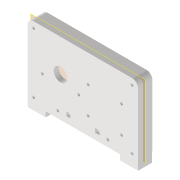
# Autodesk Inventor part: 10_Cassette_microscopy_deck
Saved by Autodesk Inventor 2022 (Build 260153000, 153)
## iProperties
Created: 2023-02-06
Part Number: 10_Cassette_microscopy_deck
Material: Generisch
Document SubType Name: Modeling
Designer: diederichbenedict
Density: 1 g/cm^3
Appearance: Vorgabe
Author: diederichbenedict
Autodesk Inventor part; units mm, degrees
ref_plane "YZ Plane" through (0, 0, 0) normal (1, 0, 0) x (0, 1, 0)
ref_plane "Arbeitsebene1" through (0, 0, 0) normal (0, 0, 1) x (1, 0, 0)
sketch "Skizze1" plane through (0, 0, 0) normal (0, 0, 1) x (1, 0, 0)
  line L0 (79.0515, 12.2449) -> (82.2341, -2.728) projected
  arc A0 (82.2417, -2.8) -> (82.2341, -2.728) centre (81.8953, -2.8001) ccw projected
  line L1 (82.2417, -2.8) -> (94.4, -2.8) projected
  arc A1 (94.4, -2.8) -> (97.2, 0) centre (94.4, 0) ccw projected
  line L2 (97.2, 0) -> (97.2, 57.5) projected
  arc A2 (97.2, 57.5) -> (94.4, 60.3) centre (94.4, 57.5) ccw projected
  line L3 (94.4, 60.3) -> (0, 60.3) projected
  arc A3 (0, 60.3) -> (-2.8, 57.5) centre (0, 57.5) ccw projected
  line L4 (-2.8, 57.5) -> (-2.8, 0) projected
  arc A4 (-2.8, 0) -> (0, -2.8) centre (0, 0) ccw projected
  line L5 (0, -2.8) -> (12.1583, -2.8) projected
  arc A5 (12.1659, -2.728) -> (12.1583, -2.8) centre (12.5047, -2.8001) ccw projected
  line L6 (12.1659, -2.728) -> (15.3485, 12.2449) projected
  spline S0 degree 3 poles (15.3485, 12.2449) (15.4002, 12.4886) (15.5255, 12.6991) (15.7047, 12.8442) (15.8839, 12.9893) (16.1159, 13.0681) (16.365, 13.0681) knots 2.565195 2.565195 2.565195 2.565195 3.141593 3.141593 3.141593 3.717991 3.717991 3.717991 3.717991 projected
  line L7 (16.365, 13.0681) -> (78.035, 13.0681) projected
  spline S1 degree 3 poles (78.035, 13.0681) (78.2841, 13.0681) (78.5161, 12.9893) (78.6953, 12.8442) (78.8745, 12.6991) (78.9998, 12.4886) (79.0515, 12.2449) knots 2.565195 2.565195 2.565195 2.565195 3.141593 3.141593 3.141593 3.717991 3.717991 3.717991 3.717991 projected
  circle A6 centre (47.2, 46) radius 2.3 projected
  line L8 (45.2128, 29.3892) -> (45.2128, 34.3892) projected
  line L9 (45.2128, 34.3892) -> (47.227, 34.3892) projected
  spline S2 degree 3 poles (47.227, 34.3892) (47.2755, 34.3889) (47.3689, 34.3884) (47.5045, 34.3868) (47.6304, 34.3823) (47.7467, 34.3783) (47.8531, 34.3692) (47.9503, 34.362) (48.0382, 34.3521) (48.1418, 34.3361) (48.2622, 34.3113) (48.3982, 34.2653) (48.5271, 34.2078) (48.647, 34.1347) (48.7582, 34.0492) (48.8617, 33.9521) (48.9526, 33.8392) (49.0345, 33.7161) (49.1036, 33.5825) (49.1512, 33.4389) (49.1816, 33.2877) (49.1853, 33.1841) (49.1872, 33.1312) knots 0 0 0 0 0.054831 0.105884 0.153553 0.197457 0.237653 0.274456 0.307946 0.337788 0.393117 0.446926 0.500064 0.552657 0.605522 0.658748 0.713023 0.769236 0.826057 0.882736 0.940135 1 1 1 1 projected
  spline S3 degree 3 poles (49.1872, 33.1312) (49.1852, 33.0736) (49.1814, 32.96) (49.1456, 32.7934) (49.0886, 32.6341) (49.0082, 32.4845) (48.9096, 32.3472) (48.7931, 32.2267) (48.6602, 32.1236) (48.5604, 32.0723) (48.5101, 32.0465) knots 0 0 0 0 0.127883 0.252157 0.376787 0.502926 0.628342 0.751132 0.874457 1 1 1 1 projected
  spline S4 degree 3 poles (48.5101, 32.0465) (48.544, 32.0349) (48.611, 32.0121) (48.7069, 31.9702) (48.7968, 31.9215) (48.8806, 31.8678) (48.959, 31.8084) (49.0295, 31.7416) (49.0964, 31.671) (49.1552, 31.5932) (49.2083, 31.5118) (49.2534, 31.4256) (49.2925, 31.3367) (49.3252, 31.2441) (49.3485, 31.1473) (49.3671, 31.0475) (49.3767, 30.9439) (49.3785, 30.8739) (49.3795, 30.8385) knots 0 0 0 0 0.067041 0.132557 0.19578 0.258217 0.318868 0.379478 0.440087 0.500739 0.561785 0.621919 0.682673 0.743576 0.805446 0.868975 0.933677 1 1 1 1 projected
  spline S5 degree 3 poles (49.3795, 30.8385) (49.3775, 30.782) (49.3735, 30.6692) (49.3435, 30.5009) (49.2928, 30.3355) (49.2242, 30.1742) (49.139, 30.0221) (49.0388, 29.8833) (48.9219, 29.7624) (48.7924, 29.656) (48.6465, 29.5678) (48.4843, 29.5001) (48.3069, 29.449) (48.1819, 29.432) (48.1175, 29.4233) knots 0 0 0 0 0.081255 0.162135 0.244884 0.329397 0.413636 0.495044 0.574817 0.654649 0.735398 0.818839 0.906654 1 1 1 1 projected
  spline S6 degree 3 poles (48.1175, 29.4233) (48.0928, 29.4212) (48.0361, 29.4164) (47.9399, 29.4104) (47.8217, 29.4059) (47.6815, 29.4006) (47.5189, 29.3968) (47.3342, 29.3942) (47.1272, 29.3908) (46.982, 29.3897) (46.9055, 29.3892) knots 0 0 0 0 0.061321 0.140766 0.238316 0.354022 0.487867 0.640687 0.810851 1 1 1 1 projected
  line L10 (46.9055, 29.3892) -> (45.2128, 29.3892) projected
  circle A7 centre (68.575, 31.8892) radius 6.4815 projected
  circle A8 centre (25.825, 31.8892) radius 6.4815 projected
  line L11 (44.025, 27.3892) -> (44.025, 15.8892) projected
  arc A9 (41.825, 13.6892) -> (44.025, 15.8892) centre (41.825, 15.8892) ccw projected
  line L12 (41.825, 13.6892) -> (9.825, 13.6892) projected
  arc A10 (7.625, 15.8892) -> (9.825, 13.6892) centre (9.825, 15.8892) ccw projected
  line L13 (7.625, 15.8892) -> (7.625, 47.8892) projected
  arc A11 (9.825, 50.0892) -> (7.625, 47.8892) centre (9.825, 47.8892) ccw projected
  line L14 (9.825, 50.0892) -> (41.825, 50.0892) projected
  arc A12 (44.025, 47.8892) -> (41.825, 50.0892) centre (41.825, 47.8892) ccw projected
  line L15 (44.025, 47.8892) -> (44.025, 36.3892) projected
  arc A13 (41.825, 34.1892) -> (44.025, 36.3892) centre (41.825, 36.3892) ccw projected
  line L16 (41.825, 34.1892) -> (33.4237, 34.1892) projected
  arc A14 (32.3338, 34.8872) -> (33.4237, 34.1892) centre (33.4237, 35.3892) ccw projected
  arc A15 (32.3338, 34.8872) -> (19.2006, 34.6222) centre (25.825, 31.8892) ccw projected
  arc A16 (18.5535, 34.1892) -> (19.2006, 34.6222) centre (18.5535, 34.8892) ccw projected
  line L17 (18.5535, 34.1892) -> (18.3962, 34.1892) projected
  arc A17 (18.3962, 34.1892) -> (17.5962, 33.3892) centre (18.3962, 33.3892) ccw projected
  line L18 (17.5962, 33.3892) -> (17.5962, 30.3892) projected
  arc A18 (17.5962, 30.3892) -> (18.3962, 29.5892) centre (18.3962, 30.3892) ccw projected
  line L19 (18.3962, 29.5892) -> (18.5535, 29.5892) projected
  arc A19 (19.2006, 29.1562) -> (18.5535, 29.5892) centre (18.5535, 28.8892) ccw projected
  arc A20 (19.2006, 29.1562) -> (32.3338, 28.8912) centre (25.825, 31.8892) ccw projected
  arc A21 (33.4237, 29.5892) -> (32.3338, 28.8912) centre (33.4237, 28.3892) ccw projected
  line L20 (33.4237, 29.5892) -> (41.825, 29.5892) projected
  arc A22 (44.025, 27.3892) -> (41.825, 29.5892) centre (41.825, 27.3892) ccw projected
  line L21 (84.575, 13.6892) -> (52.575, 13.6892) projected
  arc A23 (50.375, 15.8892) -> (52.575, 13.6892) centre (52.575, 15.8892) ccw projected
  line L22 (50.375, 15.8892) -> (50.375, 27.3892) projected
  arc A24 (52.575, 29.5892) -> (50.375, 27.3892) centre (52.575, 27.3892) ccw projected
  line L23 (52.575, 29.5892) -> (60.9763, 29.5892) projected
  arc A25 (62.0662, 28.8912) -> (60.9763, 29.5892) centre (60.9763, 28.3892) ccw projected
  arc A26 (62.0662, 28.8912) -> (75.1994, 29.1562) centre (68.575, 31.8892) ccw projected
  arc A27 (75.8465, 29.5892) -> (75.1994, 29.1562) centre (75.8465, 28.8892) ccw projected
  line L24 (75.8465, 29.5892) -> (76.0038, 29.5892) projected
  arc A28 (76.0038, 29.5892) -> (76.8038, 30.3892) centre (76.0038, 30.3892) ccw projected
  line L25 (76.8038, 30.3892) -> (76.8038, 33.3892) projected
  arc A29 (76.8038, 33.3892) -> (76.0038, 34.1892) centre (76.0038, 33.3892) ccw projected
  line L26 (76.0038, 34.1892) -> (75.8465, 34.1892) projected
  arc A30 (75.1994, 34.6222) -> (75.8465, 34.1892) centre (75.8465, 34.8892) ccw projected
  arc A31 (75.1994, 34.6222) -> (62.0662, 34.8872) centre (68.575, 31.8892) ccw projected
  arc A32 (60.9763, 34.1892) -> (62.0662, 34.8872) centre (60.9763, 35.3892) ccw projected
  line L27 (60.9763, 34.1892) -> (52.575, 34.1892) projected
  arc A33 (50.375, 36.3892) -> (52.575, 34.1892) centre (52.575, 36.3892) ccw projected
  line L28 (50.375, 36.3892) -> (50.375, 47.8892) projected
  arc A34 (52.575, 50.0892) -> (50.375, 47.8892) centre (52.575, 47.8892) ccw projected
  line L29 (52.575, 50.0892) -> (84.575, 50.0892) projected
  arc A35 (86.775, 47.8892) -> (84.575, 50.0892) centre (84.575, 47.8892) ccw projected
  line L30 (86.775, 47.8892) -> (86.775, 15.8892) projected
  arc A36 (84.575, 13.6892) -> (86.775, 15.8892) centre (84.575, 15.8892) ccw projected
  line L31 (0, 63.3) -> (94.4, 63.3)
  arc A37 (100.2, 57.5) -> (94.4, 63.3) centre (94.4, 57.5) ccw
  line L32 (100.2, 57.5) -> (100.2, 0)
  arc A38 (94.4, -5.8) -> (100.2, 0) centre (94.4, 0) ccw
  line L33 (94.4, -5.8) -> (79.8201, -5.8)
  line L34 (79.8201, -5.8) -> (76.1171, 11.6212)
  line L35 (78.035, 10.0681) -> (16.365, 10.0681)
  line L36 (18.2829, 11.6212) -> (14.5799, -5.8)
  line L37 (14.5799, -5.8) -> (0, -5.8)
  arc A39 (-5.8, 0) -> (0, -5.8) centre (0, 0) ccw
  line L38 (-5.8, 0) -> (-5.8, 57.5)
  arc A40 (0, 63.3) -> (-5.8, 57.5) centre (0, 57.5) ccw
  line L39 (12.1659, -2.728) -> (11.5129, -5.8)
  line L40 (82.2417, -2.8) -> (82.8871, -5.8)
  spline S7 degree 5 poles (76.1171, 11.6212) (76.2271, 11.0998) (76.532, 10.6219) (76.9713, 10.2662) (77.5021, 10.0673) (78.035, 10.0681) knots 0 0 0 0 0 0 1 1 1 1 1 1
  spline S8 degree 5 poles (16.365, 10.0681) (16.8979, 10.0673) (17.4287, 10.2662) (17.868, 10.6219) (18.1729, 11.0998) (18.2829, 11.6212) knots 0 0 0 0 0 0 1 1 1 1 1 1
  point P0 (12.1506, -2.8)
  dimension "d0" = 3
  constraints: 20 end point, 8 point on circle, 5 parallel, 4 centre point, 2 point on line, 15 other
  measures "d0" distance between parallel lines of L3 L31
ref_plane "Arbeitsebene2" through (4.825, 5.3892, 4.8) normal (0, 0, 1) x (1, 0, 0)
extrude "Extrusion1" add sketch "Skizze1" along normal up to surface (4.8 mm away) contours S1 L7 S0 L6 L39 L5 A4 L4 A3 L3 A2 L2 A1 L1 A0 L0 | L1 A1 L2 A2 L3 A3 L4 A4 L5 L39 L37 A39 L38 A40 L31 A37 L32 A38 L33 L40 | A5 L5 L39 | A6 | L8 L9 S2 S3 S4 S5 S6 L10 | A7 | L11 A9 L12 A10 L13 A11 L14 A12 L15 A13 L16 A14 A15 A16 L17 A17 L18 A18 L19 A19 A20 A21 L20 A22 | L21 A23 L22 A24 L23 A25 A26 A27 L24 A28 L25 A29 L26 A30 A31 A32 L27 A33 L28 A34 L29 A35 L30 A36
sketch "Skizze2" plane through (0, 63.3, 4.8) normal (0, 0, 1) x (1, 0, 0)
  circle A0 centre (8.325, -39.4108) radius 2.1 projected
  circle A1 centre (43.325, -39.4108) radius 2.1 projected
  circle A2 centre (8.325, -39.4108) radius 1.4
  circle A3 centre (43.325, -39.4108) radius 1.4
  point P0 (0, -63.3)
  dimension "d3" = 2.8
  dimension "d4" = 2.8
  constraints: 2 centre point, 2 coincident
  measures "d3" diameter of A2
  measures "d4" diameter of A3
extrude "Extrusion2" cut sketch "Skizze2" against normal blind 10 contours A2 | A3
sketch "Skizze3" plane through (0, 0, 0) normal (0, 0, -1) x (-1, 0, 0)
  line L0 (-94.4, -2.8) -> (-82.2417, -2.8) projected
  arc A0 (-82.2341, -2.728) -> (-82.2417, -2.8) centre (-81.8953, -2.8001) ccw projected
  line L1 (-82.2341, -2.728) -> (-79.0515, 12.2449) projected
  spline S0 degree 3 poles (-79.0515, 12.2449) (-78.9998, 12.4886) (-78.8745, 12.6991) (-78.6953, 12.8442) (-78.5161, 12.9893) (-78.2841, 13.0681) (-78.035, 13.0681) knots 2.565195 2.565195 2.565195 2.565195 3.141593 3.141593 3.141593 3.717991 3.717991 3.717991 3.717991 projected
  line L2 (-78.035, 13.0681) -> (-16.365, 13.0681) projected
  spline S1 degree 3 poles (-16.365, 13.0681) (-16.1159, 13.0681) (-15.8839, 12.9893) (-15.7047, 12.8442) (-15.5255, 12.6991) (-15.4002, 12.4886) (-15.3485, 12.2449) knots 2.565195 2.565195 2.565195 2.565195 3.141593 3.141593 3.141593 3.717991 3.717991 3.717991 3.717991 projected
  line L3 (-15.3485, 12.2449) -> (-12.1659, -2.728) projected
  arc A1 (-12.1583, -2.8) -> (-12.1659, -2.728) centre (-12.5047, -2.8001) ccw projected
  line L4 (-12.1583, -2.8) -> (0, -2.8) projected
  arc A2 (0, -2.8) -> (2.8, 0) centre (0, 0) ccw projected
  line L5 (2.8, 0) -> (2.8, 6.4087) projected
  line L6 (2.8, 6.4087) -> (-7.6627, 15.4837) projected
  arc A3 (-9.825, 13.6892) -> (-7.6627, 15.4837) centre (-9.825, 15.8892) ccw projected
  line L7 (-9.825, 13.6892) -> (-41.825, 13.6892) projected
  arc A4 (-44.025, 15.8892) -> (-41.825, 13.6892) centre (-41.825, 15.8892) ccw projected
  line L8 (-44.025, 15.8892) -> (-44.025, 27.3892) projected
  arc A5 (-41.825, 29.5892) -> (-44.025, 27.3892) centre (-41.825, 27.3892) ccw projected
  line L9 (-41.825, 29.5892) -> (-33.4237, 29.5892) projected
  arc A6 (-32.3338, 28.8912) -> (-33.4237, 29.5892) centre (-33.4237, 28.3892) ccw projected
  arc A7 (-32.3338, 28.8912) -> (-32.3338, 34.8872) centre (-25.825, 31.8892) ccw projected
  arc A8 (-33.4237, 34.1892) -> (-32.3338, 34.8872) centre (-33.4237, 35.3892) ccw projected
  line L10 (-33.4237, 34.1892) -> (-41.825, 34.1892) projected
  arc A9 (-44.025, 36.3892) -> (-41.825, 34.1892) centre (-41.825, 36.3892) ccw projected
  line L11 (-44.025, 36.3892) -> (-44.025, 47.8892) projected
  arc A10 (-41.825, 50.0892) -> (-44.025, 47.8892) centre (-41.825, 47.8892) ccw projected
  line L12 (-41.825, 50.0892) -> (-9.825, 50.0892) projected
  arc A11 (-7.625, 47.8892) -> (-9.825, 50.0892) centre (-9.825, 47.8892) ccw projected
  line L13 (-7.625, 47.8892) -> (-7.625, 17.9661) projected
  line L14 (-7.625, 17.9661) -> (2.8, 8.9238) projected
  line L15 (2.8, 8.9238) -> (2.8, 57.5) projected
  arc A12 (2.8, 57.5) -> (0, 60.3) centre (0, 57.5) ccw projected
  line L16 (0, 60.3) -> (-94.4, 60.3) projected
  arc A13 (-94.4, 60.3) -> (-97.2, 57.5) centre (-94.4, 57.5) ccw projected
  line L17 (-97.2, 57.5) -> (-97.2, 0) projected
  arc A14 (-97.2, 0) -> (-94.4, -2.8) centre (-94.4, 0) ccw projected
  circle A15 centre (-25.825, 31.8892) radius 6.4815 projected
  circle A16 centre (-68.575, 31.8892) radius 6.4815 projected
  arc A17 (-75.0838, 28.8912) -> (-76.1737, 29.5892) centre (-76.1737, 28.3892) ccw projected
  arc A18 (-75.0838, 28.8912) -> (-62.0662, 28.8912) centre (-68.575, 31.8892) ccw projected
  arc A19 (-60.9763, 29.5892) -> (-62.0662, 28.8912) centre (-60.9763, 28.3892) ccw projected
  line L18 (-60.9763, 29.5892) -> (-52.575, 29.5892) projected
  arc A20 (-50.375, 27.3892) -> (-52.575, 29.5892) centre (-52.575, 27.3892) ccw projected
  line L19 (-50.375, 27.3892) -> (-50.375, 15.8892) projected
  arc A21 (-52.575, 13.6892) -> (-50.375, 15.8892) centre (-52.575, 15.8892) ccw projected
  line L20 (-52.575, 13.6892) -> (-84.575, 13.6892) projected
  arc A22 (-86.775, 15.8892) -> (-84.575, 13.6892) centre (-84.575, 15.8892) ccw projected
  line L21 (-86.775, 15.8892) -> (-86.775, 47.8892) projected
  arc A23 (-84.575, 50.0892) -> (-86.775, 47.8892) centre (-84.575, 47.8892) ccw projected
  line L22 (-84.575, 50.0892) -> (-52.575, 50.0892) projected
  arc A24 (-50.375, 47.8892) -> (-52.575, 50.0892) centre (-52.575, 47.8892) ccw projected
  line L23 (-50.375, 47.8892) -> (-50.375, 36.3892) projected
  arc A25 (-52.575, 34.1892) -> (-50.375, 36.3892) centre (-52.575, 36.3892) ccw projected
  line L24 (-52.575, 34.1892) -> (-60.9763, 34.1892) projected
  arc A26 (-62.0662, 34.8872) -> (-60.9763, 34.1892) centre (-60.9763, 35.3892) ccw projected
  arc A27 (-62.0662, 34.8872) -> (-75.0838, 34.8872) centre (-68.575, 31.8892) ccw projected
  arc A28 (-76.1737, 34.1892) -> (-75.0838, 34.8872) centre (-76.1737, 35.3892) ccw projected
  line L25 (-76.1737, 34.1892) -> (-76.5038, 34.1892) projected
  arc A29 (-76.5038, 34.1892) -> (-76.8038, 33.8892) centre (-76.5038, 33.8892) ccw projected
  line L26 (-76.8038, 33.8892) -> (-76.8038, 29.8892) projected
  arc A30 (-76.8038, 29.8892) -> (-76.5038, 29.5892) centre (-76.5038, 29.8892) ccw projected
  line L27 (-76.5038, 29.5892) -> (-76.1737, 29.5892) projected
  circle A31 centre (-47.2, 46) radius 2.3 projected
  circle A32 centre (-94.35, 57.6) radius 2.265 projected
  circle A33 centre (-82.2, 10) radius 2.265 projected
  circle A34 centre (-0.05, 57.6) radius 2.265 projected
  circle A35 centre (-12.2, 10) radius 2.265 projected
  line L28 (-46.6952, 34.3892) -> (-44.7962, 29.3892) projected
  line L29 (-44.7962, 29.3892) -> (-45.8158, 29.3892) projected
  line L30 (-45.8158, 29.3892) -> (-46.2375, 30.543) projected
  line L31 (-46.2375, 30.543) -> (-48.1565, 30.543) projected
  line L32 (-48.1565, 30.543) -> (-48.5782, 29.3892) projected
  line L33 (-48.5782, 29.3892) -> (-49.6038, 29.3892) projected
  line L34 (-49.6038, 29.3892) -> (-47.7138, 34.3892) projected
  line L35 (-47.7138, 34.3892) -> (-46.6952, 34.3892) projected
  circle A36 centre (-43.325, 23.8892) radius 1.4 projected
  circle A37 centre (-8.325, 23.8892) radius 1.4 projected
  line L36 (-12.1659, -2.728) -> (-15.3485, 12.2449) projected
  arc A38 (-12.1583, -2.8) -> (-12.1659, -2.728) centre (-12.5047, -2.8001) ccw projected
  line L37 (-12.1506, -2.8) -> (-12.1583, -2.8) projected
  line L38 (-11.5129, -5.8) -> (-12.1506, -2.8) projected
  line L39 (0, -5.8) -> (-11.5129, -5.8) projected
  arc A39 (0, -5.8) -> (5.8, 0) centre (0, 0) ccw projected
  line L40 (5.8, 57.5) -> (5.8, 0) projected
  arc A40 (5.8, 57.5) -> (0, 63.3) centre (0, 57.5) ccw projected
  line L41 (-94.4, 63.3) -> (0, 63.3) projected
  arc A41 (-94.4, 63.3) -> (-100.2, 57.5) centre (-94.4, 57.5) ccw projected
  line L42 (-100.2, 0) -> (-100.2, 57.5) projected
  arc A42 (-100.2, 0) -> (-94.4, -5.8) centre (-94.4, 0) ccw projected
  line L43 (-82.8871, -5.8) -> (-94.4, -5.8) projected
  line L44 (-82.2417, -2.8) -> (-82.8871, -5.8) projected
  arc A43 (-82.2341, -2.728) -> (-82.2417, -2.8) centre (-81.8953, -2.8001) ccw projected
  line L45 (-79.0515, 12.2449) -> (-82.2341, -2.728) projected
  line L46 (-16.365, 13.0681) -> (-78.035, 13.0681) projected
  circle A44 centre (-25.825, 31.8892) radius 6.4815 projected
  line L47 (-94.4, 60.8) -> (0, 60.8)
  arc A45 (3.3, 57.5) -> (0, 60.8) centre (0, 57.5) ccw
  line L48 (3.3, 57.5) -> (3.3, 7.8283)
  line L49 (3.3, 7.8283) -> (-8.125, 17.7379)
  line L50 (-8.125, 17.7379) -> (-8.125, 47.8892)
  arc A46 (-8.125, 47.8892) -> (-9.825, 49.5892) centre (-9.825, 47.8892) ccw
  line L51 (-9.825, 49.5892) -> (-41.825, 49.5892)
  arc A47 (-41.825, 49.5892) -> (-43.525, 47.8892) centre (-41.825, 47.8892) ccw
  line L52 (-43.525, 47.8892) -> (-43.525, 36.3892)
  arc A48 (-43.525, 36.3892) -> (-41.825, 34.6892) centre (-41.825, 36.3892) ccw
  line L53 (-41.825, 34.6892) -> (-33.4237, 34.6892)
  arc A49 (-33.4237, 34.6892) -> (-32.7879, 35.0963) centre (-33.4237, 35.3892) ccw
  arc A50 (-32.7879, 28.6821) -> (-32.7879, 35.0963) centre (-25.825, 31.8892) ccw
  arc A51 (-32.7879, 28.6821) -> (-33.4237, 29.0892) centre (-33.4237, 28.3892) ccw
  line L54 (-33.4237, 29.0892) -> (-41.825, 29.0892)
  arc A52 (-41.825, 29.0892) -> (-43.525, 27.3892) centre (-41.825, 27.3892) ccw
  line L55 (-43.525, 27.3892) -> (-43.525, 15.8892)
  arc A53 (-43.525, 15.8892) -> (-41.825, 14.1892) centre (-41.825, 15.8892) ccw
  line L56 (-41.825, 14.1892) -> (-9.825, 14.1892)
  arc A54 (-9.825, 14.1892) -> (-8.3585, 16.7491) centre (-9.825, 15.8892) ccw
  line L57 (-8.3585, 16.7491) -> (3.3, 6.6369)
  line L58 (3.3, 6.6369) -> (3.3, 0)
  arc A55 (0, -3.3) -> (3.3, 0) centre (0, 0) ccw
  line L59 (0, -3.3) -> (-12.5554, -3.3)
  line L60 (-12.5554, -3.3) -> (-15.8375, 12.141)
  line L61 (-16.365, 12.5681) -> (-78.035, 12.5681)
  line L62 (-78.5625, 12.141) -> (-81.8446, -3.3)
  line L63 (-81.8446, -3.3) -> (-94.4, -3.3)
  arc A56 (-97.7, 0) -> (-94.4, -3.3) centre (-94.4, 0) ccw
  line L64 (-97.7, 0) -> (-97.7, 57.5)
  arc A57 (-94.4, 60.8) -> (-97.7, 57.5) centre (-94.4, 57.5) ccw
  line L65 (3.3, 7.8283) -> (3.3, 6.6369)
  spline S2 degree 4 poles (-15.8375, 12.141) (-15.8569, 12.2316) (-15.892, 12.3186) (-16.0028, 12.4761) (-16.1799, 12.5517) (-16.2723, 12.5679) (-16.365, 12.5681) knots 0 0 0 0 0 0.5 0.5 1 1 1 1 1
  spline S3 degree 4 poles (-78.035, 12.5681) (-78.1277, 12.5679) (-78.2201, 12.5517) (-78.3972, 12.4761) (-78.508, 12.3186) (-78.5431, 12.2316) (-78.5625, 12.141) knots 0 0 0 0 0 0.5 0.5 1 1 1 1 1
  point P0 (-82.3493, -3.3)
  point P1 (-8.125, 22.5036)
  point P2 (-8.125, 25.2748)
  point P3 (-43.525, 25.2748)
  point P4 (-43.525, 22.5036)
  point P5 (-12.0443, -3.3)
  dimension "d7" = 0.5
  constraints: 38 end point, 26 point on circle, 13 centre point, 4 parallel, 1 vertical, 36 other
  measures "d7" distance between parallel lines of L16 L47
extrude "Extrusion3" add sketch "Skizze3" along normal blind 9 contours L44 L43 A42 L42 A41 L41 A40 L40 A39 L39 L38 L59 A55 L58 L65 L48 A45 L47 A57 L64 A56 L63
sketch "Skizze4" plane through (0, 0, 0) normal (0, 0, -1) x (-1, 0, 0)
  circle A0 centre (-68.575, 31.8892) radius 5.5 projected
  line L0 (-69.7138, 35.7963) -> (-71.0519, 35.1184) projected
  circle A1 centre (-68.575, 31.8892) radius 3.75
  point P0 (0, 0)
  dimension "d10" = 7.5
  constraints: 1 centre point, 1 coincident
  measures "d10" diameter of A1
extrude "Extrusion4" add sketch "Skizze4" along normal up to surface (9 mm away) draft -3 contours A1
sketch "Skizze5" plane through (0, 63.3, 4.8) normal (0, 0, 1) x (1, 0, 0)
  circle A0 centre (43.325, -39.4108) radius 1.4 projected
  circle A1 centre (8.325, -39.4108) radius 1.4 projected
  line L0 (15.3485, -51.0551) -> (12.1659, -66.028) projected
  spline S0 degree 3 poles (16.365, -50.2319) (16.1159, -50.2319) (15.8839, -50.3107) (15.7047, -50.4558) (15.5255, -50.6009) (15.4002, -50.8114) (15.3485, -51.0551) knots 0 0 0 0 0.5 0.5 0.5 1 1 1 1 projected
  line L1 (78.035, -50.2319) -> (16.365, -50.2319) projected
  spline S1 degree 3 poles (79.0515, -51.0551) (78.9998, -50.8114) (78.8745, -50.6009) (78.6953, -50.4558) (78.5161, -50.3107) (78.2841, -50.2319) (78.035, -50.2319) knots 0 0 0 0 0.5 0.5 0.5 1 1 1 1 projected
  line L2 (82.2341, -66.028) -> (79.0515, -51.0551) projected
  arc A2 (82.2417, -66.1) -> (82.2341, -66.028) centre (81.8953, -66.1001) ccw projected
  line L3 (82.8871, -69.1) -> (82.2417, -66.1) projected
  line L4 (94.4, -69.1) -> (82.8871, -69.1) projected
  arc A3 (94.4, -69.1) -> (100.2, -63.3) centre (94.4, -63.3) ccw projected
  line L5 (100.2, -5.8) -> (100.2, -63.3) projected
  arc A4 (100.2, -5.8) -> (94.4, 0) centre (94.4, -5.8) ccw projected
  line L6 (0, 0) -> (94.4, 0) projected
  arc A5 (0, 0) -> (-5.8, -5.8) centre (0, -5.8) ccw projected
  line L7 (-5.8, -63.3) -> (-5.8, -5.8) projected
  arc A6 (-5.8, -63.3) -> (0, -69.1) centre (0, -63.3) ccw projected
  line L8 (11.5129, -69.1) -> (0, -69.1) projected
  line L9 (12.1506, -66.1) -> (11.5129, -69.1) projected
  line L10 (12.1583, -66.1) -> (12.1506, -66.1) projected
  arc A7 (12.1659, -66.028) -> (12.1583, -66.1) centre (12.5047, -66.1001) ccw projected
  circle A8 centre (25.825, -31.4108) radius 6.4815 projected
  circle A9 centre (71.2, -62.7) radius 2.45 projected
  circle A10 centre (23.2, -62.7) radius 2.45 projected
  line L11 (82.8871, -69.1) -> (82.2417, -66.1) projected
  line L12 (82.8871, -69.1) -> (11.5129, -69.1)
  circle A11 centre (71.2, -62.7) radius 1.4
  circle A12 centre (23.2, -62.7) radius 1.4
  point P0 (0, -63.3)
  dimension "d15" = 2.8
  dimension "d16" = 2.8
  constraints: 2 centre point, 2 coincident, 2 end point, 1 horizontal, 2 other
  measures "d15" diameter of A11
  measures "d16" diameter of A12
extrude "Extrusion5" add sketch "Skizze5" against normal blind 2.5 contours S0 L1 S1 L2 A2 L3 L12 L9 L10 A7 L0 | A9 | A10
sketch "Skizze6" plane through (0, 0, -9) normal (0, 0, -1) x (-1, 0, 0)
  arc A0 (0, -5.8) -> (5.8, 0) centre (0, 0) ccw projected
  line L0 (5.8, 0) -> (5.8, 57.5) projected
  arc A1 (5.8, 57.5) -> (0, 63.3) centre (0, 57.5) ccw projected
  line L1 (0, 63.3) -> (-94.4, 63.3) projected
  arc A2 (-94.4, 63.3) -> (-100.2, 57.5) centre (-94.4, 57.5) ccw projected
  line L2 (-100.2, 57.5) -> (-100.2, 0) projected
  arc A3 (-100.2, 0) -> (-94.4, -5.8) centre (-94.4, 0) ccw projected
  line L3 (-94.4, -5.8) -> (-82.8871, -5.8) projected
  line L4 (-82.8871, -5.8) -> (-82.3493, -3.3) projected
  line L5 (-82.3493, -3.3) -> (-94.4, -3.3) projected
  arc A4 (-97.7, 0) -> (-94.4, -3.3) centre (-94.4, 0) ccw projected
  line L6 (-97.7, 0) -> (-97.7, 57.5) projected
  arc A5 (-94.4, 60.8) -> (-97.7, 57.5) centre (-94.4, 57.5) ccw projected
  line L7 (-94.4, 60.8) -> (0, 60.8) projected
  arc A6 (3.3, 57.5) -> (0, 60.8) centre (0, 57.5) ccw projected
  line L8 (3.3, 57.5) -> (3.3, 0) projected
  arc A7 (0, -3.3) -> (3.3, 0) centre (0, 0) ccw projected
  line L9 (0, -3.3) -> (-12.0443, -3.3) projected
  line L10 (-12.0443, -3.3) -> (-11.5129, -5.8) projected
  line L11 (-11.5129, -5.8) -> (0, -5.8) projected
  line L12 (-98.7, 16.9282) -> (4.3, 16.9282)
  line L13 (4.3, 16.9282) -> (4.3, 1.9282)
  line L14 (4.3, 1.9282) -> (-98.7, 1.9282)
  line L15 (-98.7, 1.9282) -> (-98.7, 16.9282)
  line L16 (-98.7, 16.9282) -> (4.3, 1.9282) construction
  line L17 (4.3, 16.9282) -> (-98.7, 1.9282) construction
  point P0 (-47.2, 9.4282)
  dimension "d17" = 103
  dimension "d18" = 15
  constraints: 12 end point, 2 midpoint, 2 parallel, 1 horizontal, 1 perpendicular
  measures "d17" distance of L13.end L14.end
  measures "d18" distance of L12.end L13.end
extrude "Extrusion6" cut sketch "Skizze6" against normal blind 7 contours L14 L6 L12 L8 | L8 L12 L13 L14 | L14 L15 L12 L6
sketch "Skizze7" plane through (0, -5.8, 4.8) normal (0, 0, 1) x (1, 0, 0)
  circle A0 centre (71.2, 6.4) radius 2.45 projected
  circle A1 centre (23.2, 6.4) radius 2.45 projected
  line L0 (31.2712, 9.4) -> (31.2712, 6.45) projected
  line L1 (35.3, 7.5) -> (35.3, 6.45) projected
  arc A2 (35.3, 7.5) -> (36.2, 7.5) centre (35.75, 7.5) ccw projected
  line L2 (36.2, 7.5) -> (36.2, 7.15) projected
  arc A3 (34.2, 5.15) -> (36.2, 7.15) centre (34.2, 7.15) ccw projected
  line L3 (34.2, 5.15) -> (32.2, 5.15) projected
  arc A4 (30.2, 7.15) -> (32.2, 5.15) centre (32.2, 7.15) ccw projected
  line L4 (30.2, 7.15) -> (30.2, 7.5) projected
  arc A5 (30.2, 7.5) -> (31.1, 7.5) centre (30.65, 7.5) ccw projected
  line L5 (31.1, 6.45) -> (31.1, 7.5) projected
  arc A6 (31.1, 6.45) -> (31.5, 6.05) centre (31.5, 6.45) ccw projected
  line L6 (34.9, 6.05) -> (31.5, 6.05) projected
  arc A7 (34.9, 6.05) -> (35.3, 6.45) centre (34.9, 6.45) ccw projected
  spline S0 degree 3 poles (77.3571, 17.6845) (77.5232, 17.6845) (77.6778, 17.632) (77.7973, 17.5353) (77.9167, 17.4385) (78.0003, 17.2982) (78.0348, 17.1358) knots 2.565195 2.565195 2.565195 2.565195 3.141593 3.141593 3.141593 3.717991 3.717991 3.717991 3.717991 projected
  line L7 (78.0348, 17.1358) -> (81.0394, 3) projected
  line L8 (81.0394, 3) -> (13.3606, 3) projected
  line L9 (13.3606, 3) -> (16.3652, 17.1358) projected
  spline S1 degree 3 poles (16.3652, 17.1358) (16.3997, 17.2982) (16.4833, 17.4385) (16.6027, 17.5353) (16.7222, 17.632) (16.8768, 17.6845) (17.0429, 17.6845) knots 2.565195 2.565195 2.565195 2.565195 3.141593 3.141593 3.141593 3.717991 3.717991 3.717991 3.717991 projected
  line L10 (17.0429, 17.6845) -> (77.3571, 17.6845) projected
  circle A8 centre (47.2, 13.2912) radius 2.265 projected
  circle A9 centre (71.2, 6.4) radius 2.45 projected
  arc A10 (63.4, 9.4) -> (62.9, 9.9) centre (62.9, 9.4) ccw projected
  line L11 (62.9, 9.9) -> (59.5, 9.9) projected
  arc A11 (59.5, 9.9) -> (59, 9.4) centre (59.5, 9.4) ccw projected
  line L12 (59, 9.4) -> (59, 6.45) projected
  arc A12 (59, 6.45) -> (59.5, 5.95) centre (59.5, 6.45) ccw projected
  line L13 (59.5, 5.95) -> (62.9, 5.95) projected
  arc A13 (62.9, 5.95) -> (63.4, 6.45) centre (62.9, 6.45) ccw projected
  line L14 (63.4, 6.45) -> (63.4, 9.4) projected
  arc A14 (35.1288, 9.4) -> (34.6288, 9.9) centre (34.6288, 9.4) ccw projected
  line L15 (34.6288, 9.9) -> (31.7712, 9.9) projected
  arc A15 (31.7712, 9.9) -> (31.2712, 9.4) centre (31.7712, 9.4) ccw projected
  line L16 (31.2712, 9.4) -> (31.2712, 6.45) projected
  arc A16 (31.2712, 6.45) -> (31.7712, 5.95) centre (31.7712, 6.45) ccw projected
  line L17 (31.7712, 5.95) -> (34.6288, 5.95) projected
  arc A17 (34.6288, 5.95) -> (35.1288, 6.45) centre (34.6288, 6.45) ccw projected
  line L18 (35.1288, 6.45) -> (35.1288, 9.4) projected
  circle A18 centre (23.2, 6.4) radius 2.45 projected
  point P0 (0, 5.8)
  point P1 (34.9303, 6.0512)
  point P2 (31.4697, 6.0512)
extrude "Extrusion7" cut sketch "Skizze7" against normal blind 10 contours A15 L15 A14 L18 A17 A7 L6 A6 A16 L0 | L14 A13 L13 A12 L12 A11 L11 A10
sketch "Skizze8" plane through (0, -5.8, 4.8) normal (0, 0, 1) x (1, 0, 0)
  arc A0 (34.9303, 6.0512) -> (35.1288, 6.45) centre (34.6288, 6.45) ccw projected
  arc A1 (34.9, 6.05) -> (34.9303, 6.0512) centre (34.9, 6.45) ccw projected
  line L0 (34.9, 6.05) -> (31.5, 6.05) projected
  arc A2 (31.4697, 6.0512) -> (31.5, 6.05) centre (31.5, 6.45) ccw projected
  arc A3 (31.2712, 6.45) -> (31.4697, 6.0512) centre (31.7712, 6.45) ccw projected
  line L1 (31.2712, 6.45) -> (31.2712, 9.4) projected
  arc A4 (31.7712, 9.9) -> (31.2712, 9.4) centre (31.7712, 9.4) ccw projected
  line L2 (31.7712, 9.9) -> (34.6288, 9.9) projected
  arc A5 (35.1288, 9.4) -> (34.6288, 9.9) centre (34.6288, 9.4) ccw projected
  line L3 (35.1288, 9.4) -> (35.1288, 6.45) projected
  arc A6 (59.5, 9.9) -> (59, 9.4) centre (59.5, 9.4) ccw projected
  line L4 (59.5, 9.9) -> (62.9, 9.9) projected
  arc A7 (63.4, 9.4) -> (62.9, 9.9) centre (62.9, 9.4) ccw projected
  line L5 (63.4, 9.4) -> (63.4, 6.45) projected
  arc A8 (62.9, 5.95) -> (63.4, 6.45) centre (62.9, 6.45) ccw projected
  line L6 (62.9, 5.95) -> (59.5, 5.95) projected
  arc A9 (59, 6.45) -> (59.5, 5.95) centre (59.5, 6.45) ccw projected
  line L7 (59, 6.45) -> (59, 9.4) projected
  circle A10 centre (71.2, 6.4) radius 1.4 projected
  circle A11 centre (23.2, 6.4) radius 1.4 projected
  circle A12 centre (43.325, 29.6892) radius 1.4 projected
  circle A13 centre (8.325, 29.6892) radius 1.4 projected
  circle A14 centre (25.825, 37.6892) radius 6.4815 projected
  line L8 (94.4, 0) -> (0, 0) projected
  arc A15 (94.4, 0) -> (100.2, 5.8) centre (94.4, 5.8) ccw projected
  line L9 (100.2, 63.3) -> (100.2, 5.8) projected
  arc A16 (100.2, 63.3) -> (94.4, 69.1) centre (94.4, 63.3) ccw projected
  line L10 (0, 69.1) -> (94.4, 69.1) projected
  arc A17 (0, 69.1) -> (-5.8, 63.3) centre (0, 63.3) ccw projected
  line L11 (-5.8, 5.8) -> (-5.8, 63.3) projected
  arc A18 (-5.8, 5.8) -> (0, 0) centre (0, 5.8) ccw projected
  line L12 (100.2, 5.8) -> (100.2, 0)
  line L13 (100.2, 0) -> (94.4, 0)
  arc A19 (-5.8, 5.8) -> (0, 0) centre (0, 5.8) ccw projected
  line L14 (-5.8, 5.8) -> (-5.8, 0)
  line L15 (-5.8, 0) -> (0, 0)
  line L16 (100.2, 0) -> (-5.8, 0)
  line L17 (-5.8, 0) -> (-5.8, -5)
  line L18 (-5.8, -5) -> (100.2, -5)
  line L19 (100.2, -5) -> (100.2, 0)
  line L20 (82.8871, 0) -> (82.2417, 3) projected
  line L21 (82.8871, 0) -> (82.8871, -5)
  line L22 (12.0443, 2.5) -> (11.5129, 0) projected
  line L23 (11.5129, 0) -> (11.5129, -5)
  point P0 (0, 5.8)
  point P1 (-5.8, 0)
  dimension "d23" = 5
  constraints: 20 end point, 5 perpendicular, 3 point on line, 3 tangent, 2 parallel, 2 vertical, 1 horizontal, 1 point on circle
  measures "d23" distance of L17.end L16.end
ref_plane "Arbeitsebene3" through (-2.8, -2.8002, -8.7) normal (0, 0, -1) x (0, 1, 0)
extrude "Extrusion8" add sketch "Skizze8" against normal up to surface (13.5 mm away) contours L13 L19 L18 L21 L8 | A15 L12 L13 | L23 L18 L17 L15 L8 | L15 L14 A18
sketch "Skizze9" plane through (82.8871, -10.8, 4.8) normal (0, -1, 0) x (1, 0, 0)
  line L0 (0, -13.5) -> (17.3129, -13.5) projected
  line L1 (17.3129, 0) -> (17.3129, -13.5) projected
  line L2 (0, 0) -> (17.3129, 0) projected
  line L3 (0, 0) -> (0, -13.5) projected
  line L4 (-88.6871, -13.5) -> (-71.3742, -13.5) projected
  line L5 (-71.3742, 0) -> (-71.3742, -13.5) projected
  line L6 (-88.6871, 0) -> (-71.3742, 0) projected
  line L7 (-88.6871, 0) -> (-88.6871, -13.5) projected
  circle A0 centre (8.6564, -6.75) radius 1.4
  circle A1 centre (-80.0307, -6.75) radius 1.4
  line L8 (29.3135, 8.35) -> (-0.6865, 8.35) projected
  arc A2 (31.8135, 5.85) -> (29.3135, 8.35) centre (29.3135, 5.85) ccw projected
  line L9 (31.8135, -24.15) -> (31.8135, 5.85) projected
  arc A3 (29.3135, -26.65) -> (31.8135, -24.15) centre (29.3135, -24.15) ccw projected
  line L10 (-0.6865, -26.65) -> (29.3135, -26.65) projected
  arc A4 (-3.1865, -24.15) -> (-0.6865, -26.65) centre (-0.6865, -24.15) ccw projected
  line L11 (-3.1865, 5.85) -> (-3.1865, -24.15) projected
  arc A5 (-0.6865, 8.35) -> (-3.1865, 5.85) centre (-0.6865, 5.85) ccw projected
  circle A6 centre (14.3135, 12.85) radius 4 projected
  line L12 (-3.9365, -25.1222) -> (-6.4865, -26.5945) projected
  line L13 (-6.4865, -26.5945) -> (-9.0365, -25.1222) projected
  line L14 (-9.0365, -25.1222) -> (-9.0365, -22.1778) projected
  line L15 (-9.0365, -22.1778) -> (-6.4865, -20.7055) projected
  line L16 (-6.4865, -20.7055) -> (-3.9365, -22.1778) projected
  line L17 (-3.9365, -22.1778) -> (-3.9365, -25.1222) projected
  line L18 (1.2857, -27.4) -> (2.758, -29.95) projected
  line L19 (2.758, -29.95) -> (1.2857, -32.5) projected
  line L20 (1.2857, -32.5) -> (-1.6588, -32.5) projected
  line L21 (-1.6588, -32.5) -> (-3.131, -29.95) projected
  line L22 (-3.131, -29.95) -> (-1.6588, -27.4) projected
  line L23 (-1.6588, -27.4) -> (1.2857, -27.4) projected
  line L24 (-3.9365, 6.8222) -> (-6.4865, 8.2945) projected
  line L25 (-3.9365, 3.8778) -> (-3.9365, 6.8222) projected
  line L26 (-6.4865, 2.4055) -> (-3.9365, 3.8778) projected
  line L27 (-9.0365, 3.8778) -> (-6.4865, 2.4055) projected
  line L28 (-9.0365, 6.8222) -> (-9.0365, 3.8778) projected
  line L29 (-6.4865, 8.2945) -> (-9.0365, 6.8222) projected
  line L30 (1.2857, 9.1) -> (2.758, 11.65) projected
  line L31 (-1.6588, 9.1) -> (1.2857, 9.1) projected
  line L32 (-3.131, 11.65) -> (-1.6588, 9.1) projected
  line L33 (-1.6588, 14.2) -> (-3.131, 11.65) projected
  line L34 (1.2857, 14.2) -> (-1.6588, 14.2) projected
  line L35 (2.758, 11.65) -> (1.2857, 14.2) projected
  line L36 (32.5635, -25.1222) -> (35.1135, -26.5945) projected
  line L37 (32.5635, -22.1778) -> (32.5635, -25.1222) projected
  line L38 (35.1135, -20.7055) -> (32.5635, -22.1778) projected
  line L39 (37.6635, -22.1778) -> (35.1135, -20.7055) projected
  line L40 (37.6635, -25.1222) -> (37.6635, -22.1778) projected
  line L41 (35.1135, -26.5945) -> (37.6635, -25.1222) projected
  line L42 (27.3412, -27.4) -> (25.869, -29.95) projected
  line L43 (30.2857, -27.4) -> (27.3412, -27.4) projected
  line L44 (31.758, -29.95) -> (30.2857, -27.4) projected
  line L45 (30.2857, -32.5) -> (31.758, -29.95) projected
  line L46 (27.3412, -32.5) -> (30.2857, -32.5) projected
  line L47 (25.869, -29.95) -> (27.3412, -32.5) projected
  line L48 (27.3412, 9.1) -> (25.869, 11.65) projected
  line L49 (25.869, 11.65) -> (27.3412, 14.2) projected
  line L50 (27.3412, 14.2) -> (30.2857, 14.2) projected
  line L51 (30.2857, 14.2) -> (31.758, 11.65) projected
  line L52 (31.758, 11.65) -> (30.2857, 9.1) projected
  line L53 (30.2857, 9.1) -> (27.3412, 9.1) projected
  line L54 (32.5635, 6.8222) -> (35.1135, 8.2945) projected
  line L55 (35.1135, 8.2945) -> (37.6635, 6.8222) projected
  line L56 (37.6635, 6.8222) -> (37.6635, 3.8778) projected
  line L57 (37.6635, 3.8778) -> (35.1135, 2.4055) projected
  line L58 (35.1135, 2.4055) -> (32.5635, 3.8778) projected
  line L59 (32.5635, 3.8778) -> (32.5635, 6.8222) projected
  circle A7 centre (36.3135, -9.15) radius 4 projected
  line L60 (-9.7698, -3.2502) -> (-10.1865, -3.2503) projected
  arc A8 (-4.4865, -4.1) -> (-9.7698, -3.2502) centre (-7.1965, -4.1) ccw projected
  line L61 (-4.4865, -14.2) -> (-4.4865, -4.1) projected
  arc A9 (-9.7698, -15.0498) -> (-4.4865, -14.2) centre (-7.1965, -14.2) ccw projected
  line L62 (-10.1865, -15.0497) -> (-9.7698, -15.0498) projected
  line L63 (-10.1865, -32.15) -> (-10.1865, -15.0497) projected
  arc A10 (-10.1865, -32.15) -> (-8.6865, -33.65) centre (-8.6865, -32.15) ccw projected
  line L64 (8.4138, -33.65) -> (-8.6865, -33.65) projected
  line L65 (8.4137, -33.2333) -> (8.4138, -33.65) projected
  arc A11 (9.2635, -27.95) -> (8.4137, -33.2333) centre (9.2635, -30.66) ccw projected
  line L66 (19.3635, -27.95) -> (9.2635, -27.95) projected
  arc A12 (20.2132, -33.2333) -> (19.3635, -27.95) centre (19.3635, -30.66) ccw projected
  line L67 (20.2132, -33.65) -> (20.2132, -33.2333) projected
  line L68 (37.3135, -33.65) -> (20.2132, -33.65) projected
  arc A13 (37.3135, -33.65) -> (38.8135, -32.15) centre (37.3135, -32.15) ccw projected
  line L69 (38.8135, -13.65) -> (38.8135, -32.15) projected
  line L70 (40.6774, -13.65) -> (38.8135, -13.65) projected
  arc A14 (41.4228, -14.3167) -> (40.6774, -13.65) centre (40.6774, -14.4) ccw projected
  arc A15 (41.4228, -14.3167) -> (44.4135, -14.15) centre (42.9135, -14.15) ccw projected
  line L71 (44.4135, -4.15) -> (44.4135, -14.15) projected
  arc A16 (44.4135, -4.15) -> (41.4228, -3.9833) centre (42.9135, -4.15) ccw projected
  arc A17 (40.6774, -4.65) -> (41.4228, -3.9833) centre (40.6774, -3.9) ccw projected
  line L72 (38.8135, -4.65) -> (40.6774, -4.65) projected
  line L73 (38.8135, 13.85) -> (38.8135, -4.65) projected
  arc A18 (38.8135, 13.85) -> (37.3135, 15.35) centre (37.3135, 13.85) ccw projected
  line L74 (18.8135, 15.35) -> (37.3135, 15.35) projected
  line L75 (18.8135, 17.2139) -> (18.8135, 15.35) projected
  arc A19 (19.4801, 17.9593) -> (18.8135, 17.2139) centre (19.5635, 17.2139) ccw projected
  arc A20 (19.4801, 17.9593) -> (19.3135, 20.95) centre (19.3135, 19.45) ccw projected
  line L76 (9.3135, 20.95) -> (19.3135, 20.95) projected
  arc A21 (9.3135, 20.95) -> (9.1468, 17.9593) centre (9.3135, 19.45) ccw projected
  arc A22 (9.8135, 17.2139) -> (9.1468, 17.9593) centre (9.0635, 17.2139) ccw projected
  line L77 (9.8135, 15.35) -> (9.8135, 17.2139) projected
  line L78 (-8.6865, 15.35) -> (9.8135, 15.35) projected
  arc A23 (-8.6865, 15.35) -> (-10.1865, 13.85) centre (-8.6865, 13.85) ccw projected
  line L79 (-10.1865, -3.2503) -> (-10.1865, 13.85) projected
  line L80 (29.3135, -24.15) -> (-0.6865, 5.85)
  line L81 (-0.6865, 5.85) -> (-0.6865, -24.15)
  line L82 (-0.6865, -24.15) -> (29.3135, 5.85)
  circle A24 centre (14.3135, -9.15) radius 1.4
  circle A25 centre (-85.6865, -9.15) radius 1.4
  point P0 (-82.8871, -4.8)
  dimension "d26" = 2.8
  dimension "d27" = 2.8
  dimension "d30" = 2.8
  dimension "d33" = 100
  constraints: 6 end point, 4 centre point, 1 horizontal, 1 midpoint, 1 perpendicular, 2 other
  measures "d26" diameter of A0
  measures "d27" diameter of A1
  measures "d30" diameter of A24
  measures "d33" distance of A24.centre A25.centre
extrude "Extrusion9" cut sketch "Skizze9" against normal blind 10 contours A24 L80 L82 | L82 L80 A24 | L82 A24 L80 | L80 A24 L82 | A0 | A1 | A25
sketch "Skizze10" plane through (0, 63.3, 4.8) normal (0, 0, 1) x (1, 0, 0)
  arc A0 (39.825, -39.4108) -> (11.825, -39.4108) centre (25.825, -39.4108) ccw projected
  line L0 (84.3122, -52.4108) -> (52.3122, -52.4108)
  line L1 (52.3122, -52.4108) -> (52.3122, -26.4108)
  line L2 (52.3122, -26.4108) -> (84.3122, -26.4108)
  line L3 (84.3122, -26.4108) -> (84.3122, -52.4108)
  line L4 (84.3122, -52.4108) -> (52.3122, -26.4108) construction
  line L5 (52.3122, -52.4108) -> (84.3122, -26.4108) construction
  point P0 (0, -63.3)
  point P1 (68.3122, -39.4108)
  dimension "d38" = 32
  dimension "d39" = 26
  constraints: 12 end point, 2 midpoint, 2 parallel, 1 horizontal, 1 perpendicular
  measures "d38" distance of L1.end L2.end
  measures "d39" distance of L0.end L1.end
hole "Bohrung1" at (84.3122, 36.8892, 4.8) at (84.3122, 10.8892, 4.8) at (52.3122, 10.8892, 4.8) at (52.3122, 36.8892, 4.8) direction (0, 0, -1) diameter 2.8 depth 14 tip angle 118
sketch "Skizze11" plane through (0, 63.3, 4.8) normal (0, 0, 1) x (1, 0, 0)
  circle A0 centre (52.3122, -52.4108) radius 1.4 projected
  circle A1 centre (84.3122, -26.4108) radius 1.4 projected
  circle A2 centre (84.3122, -52.4108) radius 1.4 projected
  circle A3 centre (52.3122, -26.4108) radius 1.4 projected
  arc A4 (34.9303, -63.0488) -> (35.1288, -62.65) centre (34.6288, -62.65) ccw projected
  arc A5 (34.9, -63.05) -> (34.9303, -63.0488) centre (34.9, -62.65) ccw projected
  line L0 (34.9, -63.05) -> (31.5, -63.05) projected
  arc A6 (31.4697, -63.0488) -> (31.5, -63.05) centre (31.5, -62.65) ccw projected
  arc A7 (31.2712, -62.65) -> (31.4697, -63.0488) centre (31.7712, -62.65) ccw projected
  line L1 (31.2712, -62.65) -> (31.2712, -59.7) projected
  arc A8 (31.7712, -59.2) -> (31.2712, -59.7) centre (31.7712, -59.7) ccw projected
  line L2 (31.7712, -59.2) -> (34.6288, -59.2) projected
  arc A9 (35.1288, -59.7) -> (34.6288, -59.2) centre (34.6288, -59.7) ccw projected
  line L3 (35.1288, -59.7) -> (35.1288, -62.65) projected
  arc A10 (59.5, -59.2) -> (59, -59.7) centre (59.5, -59.7) ccw projected
  line L4 (59.5, -59.2) -> (62.9, -59.2) projected
  arc A11 (63.4, -59.7) -> (62.9, -59.2) centre (62.9, -59.7) ccw projected
  line L5 (63.4, -59.7) -> (63.4, -62.65) projected
  arc A12 (62.9, -63.15) -> (63.4, -62.65) centre (62.9, -62.65) ccw projected
  line L6 (62.9, -63.15) -> (59.5, -63.15) projected
  arc A13 (59, -62.65) -> (59.5, -63.15) centre (59.5, -62.65) ccw projected
  line L7 (59, -62.65) -> (59, -59.7) projected
  circle A14 centre (71.2, -62.7) radius 1.4 projected
  circle A15 centre (23.2, -62.7) radius 1.4 projected
  circle A16 centre (43.325, -39.4108) radius 1.4 projected
  circle A17 centre (8.325, -39.4108) radius 1.4 projected
  circle A18 centre (25.825, -31.4108) radius 6.4815 projected
  line L8 (82.8871, -69.1) -> (82.8871, -74.1) projected
  line L9 (82.8871, -74.1) -> (100.2, -74.1) projected
  line L10 (100.2, -5.8) -> (100.2, -74.1) projected
  arc A19 (100.2, -5.8) -> (94.4, 0) centre (94.4, -5.8) ccw projected
  line L11 (0, 0) -> (94.4, 0) projected
  arc A20 (0, 0) -> (-5.8, -5.8) centre (0, -5.8) ccw projected
  line L12 (-5.8, -5.8) -> (-5.8, -74.1) projected
  line L13 (-5.8, -74.1) -> (11.5129, -74.1) projected
  line L14 (11.5129, -74.1) -> (11.5129, -69.1) projected
  line L15 (82.8871, -69.1) -> (11.5129, -69.1) projected
  line L16 (0, -5.8) -> (94.4, -5.8)
  line L17 (94.4, -5.8) -> (94.4, -62.7)
  line L18 (94.4, -62.7) -> (0, -62.7)
  line L19 (0, -62.7) -> (0, -5.8)
  point P0 (0, -63.3)
  constraints: 8 end point, 2 parallel, 1 horizontal, 1 perpendicular
hole "Bohrung2" at (0, 0, 4.8) at (0, 57.5, 4.8) at (94.4, 57.5, 4.8) at (94.4, 0.6, 4.8) direction (0, 0, -1) diameter 2.8 depth 14 tip angle 118
fillet "Rundung1" radius 2 1 edges at (71.8533, 31.8892, -9)
